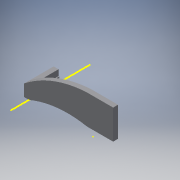
# Autodesk Inventor part: Belt_clamp
Saved by Autodesk Inventor 2019.3 (Build 233278000, 278)
## iProperties
Created: 2020-09-08
Part Number: Belt_clamp
Material: Generisch
Document SubType Name: Modeling
Designer: Nicolas Frick
Density: 1 g/cm^3
Appearance: Vorgabe
Author: Nicolas Frick
Autodesk Inventor part; units mm, degrees
ref_plane "YZ Plane" through (0, 0, 0) normal (1, 0, 0) x (0, 1, 0)
ref_plane "XZ Plane" through (0, 0, 0) normal (0, 1, 0) x (-1, 0, 0)
ref_plane "XY Plane" through (0, 0, 0) normal (0, 0, 1) x (1, 0, 0)
sketch "Skizze1" plane through (0, 0, 0) normal (0, 0, 1) x (1, 0, 0)
  circle A0 centre (-12.4383, -21.8297) radius 1 construction
  arc A1 (-32.4081, -36.5937) -> (-25.7184, -35.1283) centre (-32.4081, -20.5913) ccw construction
  arc A2 (1.6293, -36.5937) -> (-25.7184, -35.1283) centre (-13.5187, -63.3725) ccw construction
  line L0 (1.6293, -36.5937) -> (20.6293, -36.5937) construction
  line L1 (20.6293, -36.5937) -> (20.6293, 44.4063) construction
  line L2 (20.6293, 44.4063) -> (-5.8894, 44.4063) construction
  line L3 (-5.8894, 44.4063) -> (-5.8894, -7.9993) construction
  arc A3 (-5.8894, -7.9993) -> (-32.4081, -4.5888) centre (-26.7284, -65.2303) ccw construction
  line L4 (-32.4081, -4.5888) -> (-32.4081, -9.4913) construction
  arc A4 (-32.4081, -31.6913) -> (-32.4081, -9.4913) centre (-32.4081, -20.5913) ccw construction
  line L5 (-32.4081, -31.6913) -> (-32.4081, -36.5937) construction
  line L6 (-65.0681, -3.8937) -> (-65.0681, 2.1063) construction
  line L7 (-64.0708, -3.8937) -> (-64.0708, 2.1063) construction
  line L8 (-58.5255, -11.5937) -> (-77.1371, -11.5937) construction
  line L9 (-65.5908, -3.8937) -> (-64.3181, -3.8937) construction
  line L10 (-65.5908, -3.8937) -> (-64.3181, -3.8937) construction
  line L11 (-69.8894, 8.1063) -> (-64.8894, 8.1063) construction
  line L12 (-69.8894, -10.8937) -> (-69.8894, 8.1063) construction
  line L13 (-69.8894, -10.8937) -> (-64.8894, -10.8937) construction
  line L14 (-64.8894, -10.8937) -> (-64.8894, 8.1063) construction
  line L15 (-69.8894, -3.8937) -> (-64.0708, -3.8937)
  line L16 (20.6293, 2.1063) -> (20.6293, 32.1063)
  line L17 (-69.8894, 8.1063) -> (-69.8894, -3.8937)
  line L18 (-69.8894, -3.8937) -> (-64.8894, -3.8937)
  line L19 (-64.8894, 8.1063) -> (-65.0681, 8.1063)
  line L20 (-69.8894, 8.1063) -> (-69.8894, -3.8937)
  arc A5 (-5.8894, 2.1063) -> (-64.8894, -3.8937) centre (-25.526, -97.8838) ccw
  line L21 (-5.8894, 32.1063) -> (-5.8894, 2.1063)
  line L22 (-5.8894, 2.1063) -> (20.6293, 2.1063)
  line L23 (20.6293, 2.1063) -> (20.6293, 32.1063)
  line L24 (-5.8894, 2.1063) -> (-5.8894, 32.1063)
  arc A6 (-5.8894, 32.1063) -> (-69.8894, 8.1063) centre (-0.8023, -78.7928) ccw
  line L25 (-5.8894, 32.1063) -> (20.6293, 32.1063)
  point P0 (0, 0)
  point P1 (-64.3181, 2.1063)
  dimension "d1" = 30
  constraints: 22 end point, 5 point on circle, 5 point on line, 3 parallel, 2 centre point, 2 horizontal, 2 perpendicular, 1 other
  measures "d1" distance of L21.start L24.start
extrude "Extrusion1" add sketch "Skizze1" against normal blind 30
sketch "Skizze2" plane through (0, 0, -30) normal (0, 0, -1) x (-1, 0, 0)
  line L0 (-20.6293, 32.1063) -> (-20.6293, 2.1063) projected
  line L1 (5.8894, 32.1063) -> (-20.6293, 32.1063) projected
  line L2 (-20.6293, 2.1063) -> (5.8894, 2.1063) projected
  line L3 (5.8894, 44.4063) -> (5.8894, -7.9993) projected
  point P0 (0, 0)
extrude "Extrusion2" cut sketch "Skizze2" against normal blind 25
sketch "Skizze3" plane through (0, 0, -30) normal (0, 0, -1) x (-1, 0, 0)
  line L0 (5.8894, 44.4063) -> (5.8894, -7.9993) construction
  line L1 (64.8894, -10.8937) -> (69.8894, -10.8937) construction
  line L2 (64.8894, -10.8937) -> (64.8894, 8.1063) construction
  line L3 (69.8894, -10.8937) -> (69.8894, 8.1063) construction
  line L4 (64.8894, 8.1063) -> (69.8894, 8.1063) construction
  line L5 (64.4808, -3.8937) -> (64.4808, 2.1063) construction
  line L6 (64.0708, -3.8937) -> (64.0708, 2.1063) construction
  arc A0 (69.8894, 8.1063) -> (5.8894, 32.1063) centre (0.8023, -78.7928) ccw
  arc A1 (64.8894, -3.8937) -> (5.8894, 2.1063) centre (25.526, -97.8838) ccw construction
  arc A2 (64.8894, -3.8937) -> (5.8894, 2.1063) centre (25.526, -97.8838) ccw
  line L7 (69.8894, 8.1063) -> (64.8955, 8.1063)
  line L8 (64.8955, 8.1063) -> (64.8955, 2.1063)
  line L9 (64.0708, -3.555) -> (64.0708, 2.1063)
  line L10 (64.0708, 2.1063) -> (64.0708, -3.555)
  line L11 (64.0708, 2.1063) -> (64.0708, 2.207)
  line L12 (64.0708, 2.207) -> (64.8955, 2.1063)
  line L13 (69.8894, 8.1063) -> (64.8955, 8.1063)
  line L14 (64.8955, 2.1063) -> (64.0708, 2.1063)
  arc A3 (64.0708, -3.555) -> (5.8894, 2.1063) centre (25.526, -97.8838) ccw
  arc A4 (69.8894, 8.1063) -> (5.8894, 32.1063) centre (0.8023, -78.7928) ccw
  arc A5 (69.8894, 8.1063) -> (5.8894, 32.1063) centre (0.8023, -78.7928) ccw
  line L15 (5.8894, 2.1063) -> (5.8894, 32.1063)
  point P0 (0, 0)
  point P1 (60.6882, -2.2426)
  point P2 (60.6882, 14.6854)
extrude "Extrusion4" cut sketch "Skizze3" against normal blind 25
sketch "Skizze5" plane through (-69.8894, -3.8937, 0) normal (0, -1, 0) x (1, 0, 0)
  point P0 (69.8894, 0)
